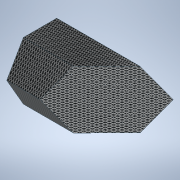
# Autodesk Inventor part: Part
Saved by Autodesk Inventor 2020 (Build 240168000, 168)
## iProperties
Created: 2019-10-28
Part Number: Part
Material: Generic
Document SubType Name: Modeling
Designer: Administrator
Density: 1 g/cm^3
Appearance: Expanded Metal 01
Author: Administrator
Autodesk Inventor part; units mm, degrees
ref_plane "YZ Plane" through (0, 0, 0) normal (1, 0, 0) x (0, 1, 0)
ref_plane "XZ Plane" through (0, 0, 0) normal (0, 1, 0) x (-1, 0, 0)
ref_plane "XY Plane" through (0, 0, 0) normal (0, 0, 1) x (1, 0, 0)
sketch "Sketch1" plane through (0, 0, 0) normal (1, 0, 0) x (0, 1, 0)
  circle A0 centre (0, 0) radius 25.4
  line L0 (0, -25.4) -> (-21.997, -12.7)
  line L1 (-21.997, -12.7) -> (-21.997, 12.7)
  line L2 (-21.997, 12.7) -> (0, 25.4)
  line L3 (0, 25.4) -> (21.997, 12.7)
  line L4 (21.997, 12.7) -> (21.997, -12.7)
  line L5 (21.997, -12.7) -> (0, -25.4)
  dimension "d0" = 50.8
  constraints: 12 end point, 2 coincident, 1 vertical alignment, 15 other
extrude "Extrusion1" add sketch "Sketch1" along normal blind 76.2 contours L4 L5 L0 L1 L2 L3
sketch "Sketch2" plane through (0, 0, 0) normal (0, 1, 0) x (-1, 0, 0)
  line L0 (0, 25.4259) -> (-25.4, 25.4)
  line L1 (0, 25.4) -> (-76.2, 25.4) projected
  line L2 (-25.4, 25.4) -> (-79.2265, -28.5365)
  line L3 (-79.2265, -28.5365) -> (-79.2893, 33.005)
  line L4 (-79.2893, 33.005) -> (-25.4, 25.4)
  point P0 (0, 0)
  dimension "d3" = 25.4
  dimension "d4" = 76.2
  dimension "d5" = 135
  constraints: 8 end point, 1 perpendicular, 1 point on line
  measures "d3" distance of L0.start L0.end
  measures "d4" distance of L0.end L2.end
  measures "d5" angle of L2 L0
extrude "Extrusion2" cut sketch "Sketch2" along normal mid plane 76.2
body "Solid1"
